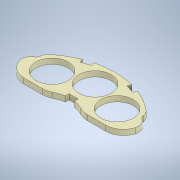
# Autodesk Inventor part: Крепление АКБ
Saved by Autodesk Inventor 2022 (Build 260153000, 153)
## iProperties
Created: 2022-05-03
Part Number: Крепление АКБ
Material: Пластик АБС
Document SubType Name: Modeling
Designer: Кочетов.А.И.
Density: 1.06 g/cm^3
Appearance: Гладкий — пепельный
Author: Кочетов.А.И.
Autodesk Inventor part; units mm, degrees
ref_plane "YZ Plane" through (0, 0, 0) normal (1, 0, 0) x (0, 1, 0)
ref_plane "XZ Plane" through (0, 0, 0) normal (0, 1, 0) x (-1, 0, 0)
ref_plane "XY Plane" through (0, 0, 0) normal (0, 0, 1) x (1, 0, 0)
sketch "Эскиз1" plane through (0, 0, 0) normal (0, 1, 0) x (-1, 0, 0)
  circle A0 centre (0, 0) radius 42
  line L0 (0, -42) -> (0, 42) construction
  circle A1 centre (18.0767, -25) radius 9
  circle A2 centre (-18.0767, -25) radius 9
  line L1 (39.598, -14) -> (-39.598, -14)
  circle A3 centre (0, -30.8507) radius 9
  circle A4 centre (0, 0) radius 30.8507 construction
  line L2 (0, 0) -> (12.9332, -39.9591) construction
  line L3 (0, 0) -> (-12.9332, -39.9591) construction
  line L4 (9.9159, -38.7553) -> (14.673, -37.2156)
  line L5 (14.673, -37.2156) -> (15.2888, -39.1184)
  line L6 (15.2888, -39.1184) -> (10.5318, -40.6581)
  line L7 (10.5318, -40.6581) -> (9.9159, -38.7553)
  line L8 (9.9159, -38.7553) -> (15.2888, -39.1184) construction
  line L9 (14.673, -37.2156) -> (10.5318, -40.6581) construction
  line L10 (-14.673, -37.2156) -> (-9.9159, -38.7553)
  line L11 (-9.9159, -38.7553) -> (-10.5318, -40.6581)
  line L12 (-10.5318, -40.6581) -> (-15.2888, -39.1184)
  line L13 (-15.2888, -39.1184) -> (-14.673, -37.2156)
  line L14 (-14.673, -37.2156) -> (-10.5318, -40.6581) construction
  line L15 (-9.9159, -38.7553) -> (-15.2888, -39.1184) construction
  line L16 (-2.5, -16.8507) -> (2.5, -16.8507)
  line L17 (2.5, -16.8507) -> (2.5, -18.8507)
  line L18 (2.5, -18.8507) -> (-2.5, -18.8507)
  line L19 (-2.5, -18.8507) -> (-2.5, -16.8507)
  line L20 (-2.5, -16.8507) -> (2.5, -18.8507) construction
  line L21 (2.5, -16.8507) -> (-2.5, -18.8507) construction
  circle A5 centre (0, 0) radius 17.0352
  circle A6 centre (0, 2) radius 44 construction
  circle A7 centre (31.1127, -29.1127) radius 2.5
  circle A8 centre (-31.1127, -29.1127) radius 2.5
  point P0 (12.6024, -38.9369)
  point P1 (-12.6024, -38.9369)
  point P2 (0, -17.8507)
  point P3 (9.7056, -14)
  point P4 (2.5, -16.8507)
  point P5 (-9.7056, -14)
  point P6 (-15.2888, -39.1184)
  point P7 (10.5318, -40.6581)
  point P8 (28.9734, -30.4063)
  point P9 (32.2615, -26.8923)
  point P10 (-32.2615, -26.8923)
  point P11 (-28.9734, -30.4063)
  dimension "d0" = 84
  dimension "d5" = 18
  dimension "d7" = 14
  dimension "d8" = 11
  dimension "d9" = 19
  dimension "d13" = 35.87
  dimension "d14" = 17.935
  dimension "d15" = 2
  dimension "d16" = 2
  dimension "d17" = 5
  dimension "d18" = 5
  dimension "d19" = 5
  dimension "d20" = 2
  dimension "d21" = 13
  dimension "d26" = 2
  dimension "d27" = 88
  dimension "d28" = 5
  dimension "d29" = 90
  constraints: 44 end point, 7 centre point, 7 midpoint, 6 parallel, 6 perpendicular, 5 coincident, 5 point on line, 4 point on circle, 3 equal radius, 1 horizontal, 1 horizontal alignment, 1 symmetric about line, 1 vertical, 14 other
  measures "d5" diameter of A1
  measures "d7" distance from line of point (0, 0) L1
  measures "d8" distance from line of L1 A2.centre
  measures "d9" distance of A1.centre A3.centre
  measures "d14" angle of L0 L2
  measures "d15" distance of L6.end L4.start
  measures "d16" distance of L10.end L11.end
  measures "d17" distance of L10.start L10.end
  measures "d18" distance of L4.start L4.end
  measures "d19" distance of L17.end L18.end
  measures "d20" distance of L16.end L17.end
  measures "d21" distance of point (0, -17.851) A3.centre
  measures "d26" distance of point (0, 0) point (0, 2)
  measures "d27" diameter of A6
  measures "d28" diameter of A8
extrude "Выдавливание2" add sketch "Эскиз1" along normal blind 3 contours L1 A5 L19 L18 L17 A0 A7 L5 L4 L7 L11 L10 L13 A8
fillet "Сопряжение1" radius 10 2 edges at (-39.598, 1.5, -14) (39.598, 1.5, -14)
fillet "Сопряжение2" radius 10 2 edges at (-9.7056, 1.5, -14) (9.7056, 1.5, -14)
fillet "Сопряжение3" radius 5 4 edges at (28.9734, 1.5, -30.4063) (32.2615, 1.5, -26.8923) (-28.9734, 1.5, -30.4063) (-32.2615, 1.5, -26.8923)
equation "\"d14\" = 0.5 * d13"
